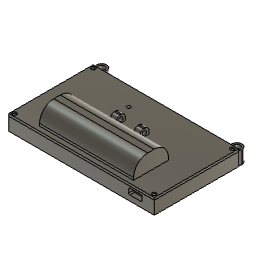
OS_EINK_CAD (Autodesk Fusion 360 design; units mm, degrees)
Autodesk Fusion 360 part; units mm, degrees
sketch "Sketch1" plane through (0, 0, 0) normal (0, 0, 1) x (1, 0, 0)
  line L0 (0, 0) -> (114, 0)
  line L1 (0, 0) -> (0, 63)
  line L2 (0, 63) -> (114, 63)
  line L3 (114, 0) -> (114, 63)
  dimension "d1" = 114
  dimension "d2" = 63
  constraint coincident L0.start L1.start
  constraint horizontal L0
  constraint perpendicular L0 L1
  constraint perpendicular L1 L2
  constraint coincident L2 L3.end
  constraint perpendicular L2 L3
  measures "d1" distance of L0.start L0.end
  measures "d2" distance of L0.start L1.end
extrude "Extrude1" add sketch "Sketch1" along normal blind 4 makes body 1
sketch "Sketch2" plane through (0, 0, 4) normal (0, 0, 1) x (-1, 0, 0)
  line L0 (0, 0) -> (-114, 0)
  line L1 (-114, 0) -> (-114, -63)
  line L2 (-114, -63) -> (0, -63)
  line L3 (0, -63) -> (0, 0)
  line L4 (-20, -3) -> (-20, -25.0318)
  line L5 (-20, -25.0318) -> (-85, -25.0318)
  line L6 (-20, -25.0318) -> (-93.9139, -25.0318)
  line L7 (-93.9139, -25.0318) -> (-93.9139, -1.7356)
  line L8 (-93.9139, -1.7356) -> (-20, -1.7356)
  line L9 (-20, -1.7356) -> (-20, -25.0318)
  constraint perpendicular L4 L5
  constraint horizontal L6
  constraint vertical L7
  constraint horizontal L8
  constraint vertical L9
extrude "Extrude2" add sketch "Sketch2" along normal blind 17 separate body contours L4 L5 L6 L7 L8 L9 makes body 2
sketch "Sketch3" plane through (0, 0, 4) normal (0, 0, 1) x (-1, 0, 0)
  line L0 (0, 0) -> (-114, 0)
  line L1 (-114, 0) -> (-114, -63)
  line L2 (-114, -63) -> (0, -63)
  line L3 (0, -63) -> (0, 0)
  line L4 (-108, -53.9996) -> (-108, -32)
  line L5 (-108, -32) -> (-14.4334, -32)
  line L6 (-14.4334, -32) -> (-14.4334, -63)
  line L7 (-14.4334, -63) -> (-108, -63)
  line L8 (-108, -63) -> (-108, -32)
  constraint horizontal L5
  constraint vertical L6
  constraint horizontal L7
  constraint vertical L8
  constraint coincident L2 L6.end
extrude "Extrude1'" add sketch "Sketch3" along normal blind 8.4 separate body contours L2 L4 L5 L6 L7 L8 makes body 3 in component "Case"
copy_body "CutPasteBodies1" bodies 3 removing the originals makes body 4
sketch "Sketch4" plane through (0, 0, 4) normal (0, 0, 1) x (-1, 0, 0)
  line L0 (0, 0) -> (-114, 0)
  line L1 (-114, 0) -> (-114, -63)
  line L2 (-114, -63) -> (0, -63)
  line L3 (0, -63) -> (0, 0)
  line L4 (-109.5, 0) -> (-109.5, -7.5)
  line L5 (-109.5, -7.5) -> (-100.2, -7.5)
  line L6 (-100.2, -7.5) -> (-100.2, 0)
  line L7 (-100.2, 0) -> (-109.5, 0)
  dimension "d19" = 7.5
  dimension "d20" = 9.3
  constraint coincident L0 L4.start
  constraint perpendicular L4 L5
  constraint coincident L0 L6.end
  constraint perpendicular L0 L6
  measures "d19" distance of L4.start L4.end
  measures "d20" distance of L4.end L5.end
extrude "Extrude3" add sketch "Sketch4" along normal blind 7.4 separate body contours L0 L4 L5 L6 L7 makes body 5
sketch "Sketch5" plane through (0, 0, 0) normal (0, 0, -1) x (1, 0, 0)
  line L0 (114, 0) -> (0, 0)
  line L1 (0, 0) -> (0, -63)
  line L2 (0, -63) -> (114, -63)
  line L3 (114, -63) -> (114, 0)
  line L4 (2.053, -1.9988) -> (111.9324, -1.9988)
  line L5 (111.9324, -1.9988) -> (111.9324, -60.7463)
  line L6 (111.9324, -60.7463) -> (2.053, -60.7463)
  line L7 (2.053, -60.7463) -> (2.053, -1.9988)
  line L8 (-3.2421, 3.0422) -> (117.6071, 3.0422)
  line L9 (117.6071, 3.0422) -> (117.6071, -66.157)
  line L10 (117.6071, -66.157) -> (-3.2421, -66.157)
  line L11 (-3.2421, -66.157) -> (-3.2421, 3.0422)
  constraint horizontal L4
  constraint vertical L5
  constraint horizontal L6
  constraint vertical L7
  constraint horizontal L8
  constraint vertical L9
  constraint horizontal L10
  constraint vertical L11
extrude "Extrude4" add sketch "Sketch5" along normal blind 2 separate body contours L0 L1 L2 L3 | L8 L9 L10 L11 makes body 6
copy_body "CutPasteBodies1'" bodies 6 removing the originals makes body 7 in component "Case"
sketch "Sketch6" plane through (0, 0, 0) normal (0, 0, 1) x (-1, 0, 0)
  line L0 (-2.053, -60.7463) -> (-111.9324, -60.7463)
  line L1 (-111.9324, -60.7463) -> (-111.9324, -1.9988)
  line L2 (-111.9324, -1.9988) -> (-2.053, -1.9988)
  line L3 (-2.053, -1.9988) -> (-2.053, -60.7463)
  line L4 (-117.6071, -66.157) -> (3.2421, -66.157)
  line L5 (3.2421, -66.157) -> (3.2421, 3.0422)
  line L6 (3.2421, 3.0422) -> (-117.6071, 3.0422)
  line L7 (-117.6071, 3.0422) -> (-117.6071, -66.157)
  line L8 (0.1598, -63.129) -> (-114.0751, -63.129)
  line L9 (-114.0751, -63.129) -> (-114.0751, 0.0707)
  line L10 (-114.0751, 0.0707) -> (0.1598, 0.0707)
  line L11 (0.1598, 0.0707) -> (0.1598, -63.129)
  line L12 (3.2421, -66.157) -> (-117.6071, -66.157)
  line L13 (-117.6071, -66.157) -> (-117.6071, 3.0422)
  line L14 (-117.6071, 3.0422) -> (3.2421, 3.0422)
  line L15 (3.2421, 3.0422) -> (3.2421, -66.157)
  constraint horizontal L8
  constraint vertical L9
  constraint horizontal L10
  constraint vertical L11
  constraint horizontal L12
  constraint vertical L13
  constraint horizontal L14
  constraint vertical L15
  constraint coincident L6.end L7.start
  constraint coincident L4.end L5.start
extrude "Extrude2'" add sketch "Sketch6" along normal blind 9 contours L4 L5 L6 L7 L12 L13 L14 L15 bodies 7 in component "Case"
sketch "Sketch7" plane through (0, 0, 9) normal (0, 0, 1) x (-1, 0, 0)
  line L0 (-114.0751, 0.0707) -> (0.1598, 0.0707)
  line L1 (0.1598, 0.0707) -> (0.1598, -63.129)
  line L2 (0.1598, -63.129) -> (-114.0751, -63.129)
  line L3 (-114.0751, -63.129) -> (-114.0751, 0.0707)
  line L4 (3.2421, 3.0422) -> (-117.6071, 3.0422)
  line L5 (-117.6071, 3.0422) -> (-117.6071, -66.157)
  line L6 (-117.6071, -66.157) -> (3.2421, -66.157)
  line L7 (3.2421, -66.157) -> (3.2421, 3.0422)
  line L8 (0.1598, -9.803) -> (1.5167, -9.803)
  line L9 (1.5167, -9.803) -> (1.5167, -57.1457)
  line L10 (1.5167, -57.1457) -> (0.1598, -57.1457)
  line L11 (0.1598, -57.1457) -> (0.1598, -9.803)
  constraint horizontal L8
  constraint vertical L9
  constraint horizontal L10
  constraint vertical L11
  constraint coincident L1 L8.start
extrude "Extrude3'" cut sketch "Sketch7" against normal blind 9 contours L1 L8 L9 L10 L11 bodies 7 in component "Case"
sketch "Sketch8" plane through (0, -3.0422, 0) normal (0, -1, 0) x (1, 0, 0)
  line L0 (-3.2421, 9) -> (-3.2421, -2)
  line L1 (-3.2421, -2) -> (117.6071, -2)
  line L2 (117.6071, -2) -> (117.6071, 9)
  line L3 (117.6071, 9) -> (-3.2421, 9)
  line L4 (96.9453, 7.5501) -> (108.2199, 7.5501)
  line L5 (108.2199, 7.5501) -> (108.2199, 2.4633)
  line L6 (108.2199, 2.4633) -> (96.9453, 2.4633)
  line L7 (96.9453, 2.4633) -> (96.9453, 7.5501)
  constraint horizontal L4
  constraint vertical L5
  constraint horizontal L6
  constraint vertical L7
extrude "Extrude4'" cut sketch "Sketch8" against normal blind 3 contours L4 L5 L6 L7 bodies 7 in component "Case"
extrude "Extrude5" cut 1 faces at (45.6223, 49.6665, 12.4) along direction (0, 0, -1) blind 4 on bodies 4 bodies 4
extrude "Extrude6" cut 1 faces at (106.4, 2.5, 11.4) along direction (0, 0, -1) blind 4 on bodies 5 bodies 5
sketch "Sketch9" plane through (0, 0, 9) normal (0, 0, 1) x (-1, 0, 0)
  line L0 (1.5167, -57.1457) -> (0.1598, -57.1457)
  line L1 (0.1598, -57.1457) -> (0.1598, -63.129)
  line L2 (0.1598, -63.129) -> (-114.0751, -63.129)
  line L3 (-114.0751, -63.129) -> (-114.0751, 0.0707)
  line L4 (-114.0751, 0.0707) -> (0.1598, 0.0707)
  line L5 (0.1598, 0.0707) -> (0.1598, -9.803)
  line L6 (0.1598, -9.803) -> (1.5167, -9.803)
  line L7 (1.5167, -9.803) -> (1.5167, -57.1457)
  line L8 (3.2421, 3.0422) -> (-117.6071, 3.0422)
  line L9 (-117.6071, 3.0422) -> (-117.6071, -66.157)
  line L10 (-117.6071, -66.157) -> (3.2421, -66.157)
  line L11 (3.2421, -66.157) -> (3.2421, 3.0422)
  circle A0 through (2.8751, 1.1502, 3) (0.6251, 2.4493, 3) (0.6251, -0.1488, 3)
  circle A1 through (-114.6218, 1.1732, 3) (-116.1218, 2.0393, 3) (-116.1218, 0.3072, 3)
  circle A2 through (-114.773, -64.2526, 3) (-116.273, -63.3865, 3) (-116.273, -65.1186, 3)
  circle A3 through (2.385, -64.4488, 3) (0.885, -63.5828, 3) (0.885, -65.3148, 3)
  point P0 (1.3751, 1.1502)
  dimension "d40" = 3
  dimension "d41" = 2
  dimension "d42" = 2
  dimension "d43" = 2
sketch "Sketch10" plane through (0, 0, 9) normal (0, 0, 1) x (-1, 0, 0)
sketch "Sketch11" plane through (0, 0, 9) normal (0, 0, 1) x (-1, 0, 0)
  line L0 (3.2373, 3.0256) -> (-117.6011, 3.0256)
  line L1 (-117.6011, 3.0256) -> (-117.6011, -66.1556)
  line L2 (-117.6011, -66.1556) -> (3.2373, -66.1556)
  line L3 (3.2373, -66.1556) -> (3.2373, 3.0256)
  constraint horizontal L0
  constraint vertical L1
  constraint horizontal L2
  constraint vertical L3
extrude "Extrude7" add sketch "Sketch11" along normal blind 3 separate body makes body 8
copy_body "CutPasteBodies2" bodies 8 removing the originals makes body 9 in component "Case"
sketch "Sketch12" plane through (0, 0, 12) normal (0, 0, 1) x (-1, 0, 0)
  line L0 (3.2373, -66.1556) -> (3.2373, 3.0256)
  line L1 (3.2373, 3.0256) -> (-117.6011, 3.0256)
  line L2 (-117.6011, 3.0256) -> (-117.6011, -66.1556)
  line L3 (-117.6011, -66.1556) -> (3.2373, -66.1556)
  line L4 (-17.965, -29.1961) -> (-97.3004, -29.1961)
  line L5 (-97.3004, -29.1961) -> (-97.3004, 0.2524)
  line L6 (-97.3004, 0.2524) -> (-17.965, 0.2524)
  line L7 (-17.965, 0.2524) -> (-17.965, -29.1961)
  constraint horizontal L4
  constraint vertical L5
  constraint horizontal L6
  constraint vertical L7
extrude "Extrude5'" add sketch "Sketch12" along normal blind 14 separate body contours L4 L5 L6 L7 makes body 10 in component "Case"
sketch "Sketch13" plane through (0, 0, 12) normal (0, 0, 1) x (1, 0, 0)
sketch "Sketch14" plane through (0, 63.129, 0) normal (0, -1, 0) x (1, 0, 0)
  line L0 (-0.1598, 0) -> (114.0751, 0)
  line L1 (114.0751, 0) -> (114.0751, 9)
  line L2 (114.0751, 9) -> (-0.1598, 9)
  line L3 (-0.1598, 9) -> (-0.1598, 0)
sketch "Sketch15" plane through (0, 66.157, 0) normal (0, 1, 0) x (-1, 0, 0)
  line L0 (-117.6071, 9) -> (-117.6071, -2)
  line L1 (-117.6071, -2) -> (3.2421, -2)
  line L2 (3.2421, -2) -> (3.2421, 9)
  line L3 (3.2421, 9) -> (-117.6071, 9)
sketch "Sketch16" plane through (0, 66.157, 0) normal (0, 1, 0) x (-1, 0, 0)
  line L0 (-94.6954, 3.5982) -> (-47.0974, 3.5982)
  line L1 (-47.0974, 3.5982) -> (-47.0974, 0.7193)
  line L2 (-47.0974, 0.7193) -> (-94.6954, 0.7193)
  line L3 (-94.6954, 0.7193) -> (-94.6954, 3.5982)
  constraint horizontal L0
  constraint vertical L1
  constraint horizontal L2
  constraint vertical L3
sketch "Sketch18" plane through (0, 0, 9) normal (0, 0, 1) x (-1, 0, 0)
  line L0 (1.5167, -57.1457) -> (0.1598, -57.1457)
  line L1 (0.1598, -57.1457) -> (0.1598, -63.129)
  line L2 (0.1598, -63.129) -> (-114.0751, -63.129)
  line L3 (-114.0751, -63.129) -> (-114.0751, 0.0707)
  line L4 (-114.0751, 0.0707) -> (0.1598, 0.0707)
  line L5 (0.1598, 0.0707) -> (0.1598, -9.803)
  line L6 (0.1598, -9.803) -> (1.5167, -9.803)
  line L7 (1.5167, -9.803) -> (1.5167, -57.1457)
  line L8 (3.2421, 3.0422) -> (-117.6071, 3.0422)
  line L9 (-117.6071, 3.0422) -> (-117.6071, -66.157)
  line L10 (-117.6071, -66.157) -> (3.2421, -66.157)
  line L11 (3.2421, -66.157) -> (3.2421, 3.0422)
  line L12 (-96.1619, -63.129) -> (-45.1217, -63.129)
  line L13 (-45.1217, -63.129) -> (-45.1217, -64.3836)
  line L14 (-45.1217, -64.3836) -> (-96.1619, -64.3836)
  line L15 (-96.1619, -64.3836) -> (-96.1619, -63.129)
  constraint horizontal L12
  constraint vertical L13
  constraint horizontal L14
  constraint vertical L15
  constraint coincident L2 L12.start
extrude "Extrude10" cut sketch "Sketch18" against normal blind 9 contours L2 L12 L13 L14 L15 bodies 7 in component "Case"
extrude "Extrude11" cut 1 faces at (77.3217, 20.0348, 9) along direction (0, 0, 1) blind 1 on bodies 9 bodies 9 10 in component "Case"
move_body "Move1" bodies 10 9 to x (1, 0, 0) y (0, 1, 0) z (0, 0, 1) at (0, 0, -1) in component "Case"
fillet "Fillet3" radius 12 1 edges at (57.6327, -0.2524, 25) on bodies 10 in component "Case"
fillet "Fillet4" radius 12 1 edges at (57.6327, 29.1961, 25) on bodies 10 in component "Case"
shell "Shell2" thickness 1 removed faces 1 at (44.4101, 19.3799, 11) on bodies 10 in component "Case"
sketch "Sketch19" plane through (0, 0, 11) normal (0, 0, -1) x (1, 0, 0)
  line L0 (18.965, -28.1961) -> (18.965, -0.7476)
  line L1 (18.965, -0.7476) -> (96.3004, -0.7476)
  line L2 (96.3004, -0.7476) -> (96.3004, -28.1961)
  line L3 (96.3004, -28.1961) -> (18.965, -28.1961)
  line L4 (97.3004, 0.2524) -> (17.965, 0.2524)
  line L5 (17.965, 0.2524) -> (17.965, -29.1961)
  line L6 (17.965, -29.1961) -> (97.3004, -29.1961)
  line L7 (97.3004, -29.1961) -> (97.3004, 0.2524)
  line L8 (18.965, -28.1961) -> (96.3004, -28.1961)
  line L9 (96.3004, -28.1961) -> (96.3004, -0.7476)
  line L10 (96.3004, -0.7476) -> (18.965, -0.7476)
  line L11 (18.965, -0.7476) -> (18.965, -28.1961)
  constraint horizontal L8
  constraint vertical L9
  constraint horizontal L10
  constraint vertical L11
  constraint coincident L1.end L2.start
  constraint coincident L0.start L3.end
extrude "Extrude12" cut sketch "Sketch19" along normal blind 44 contours L0 L1 L2 L3 L8 L9 L10 L11 bodies 9 in component "Case"
extrude "Extrude13" add 1 faces at (44.7434, 28.8628, 11) along direction (0, 0, -1) blind 0.1 on bodies 10 bodies 10 9 in component "Case"
extrude "Extrude14" add 1 faces at (117.6071, 43.0906, 5.3333) along direction (1, 0, 0) blind 1 on bodies 7 bodies 7 in component "Case"
extrude "Extrude15" add sketch "Sketch15" along normal blind 1 bodies 7 in component "Case"
extrude "Extrude16" add 1 faces at (117.9404, 66.157, 5.3333) along direction (0, 1, 0) blind 1 on bodies 7 bodies 7 in component "Case"
extrude "Extrude17" add 1 faces at (30.1537, -3.0422, 3.1544) along direction (0, -1, 0) blind 1 on bodies 7 bodies 7 in component "Case"
extrude "Extrude19" add 1 faces at (-3.2421, 19.6909, 5.3333) along direction (-1, 0, 0) blind 1 on bodies 7 bodies 7 in component "Case"
extrude "Extrude20" add 1 faces at (77.3217, 66.1556, 9.6667) along direction (0, 1, 0) blind 1 on bodies 10 bodies 10 in component "Case"
extrude "Extrude21" add 1 faces at (-3.2373, 43.7618, 10.3333) along direction (-1, 0, 0) blind 1 on bodies 10 bodies 10 in component "Case"
extrude "Extrude22" add 1 faces at (36.3755, -3.0256, 10.3333) along direction (0, -1, 0) blind 1 on bodies 10 bodies 10 in component "Case"
extrude "Extrude23" add 1 faces at (117.6011, 19.7014, 10.3333) along direction (1, 0, 0) blind 1 on bodies 10 bodies 10 in component "Case"
hole "Hole2" at (41.6318, 51.3598, 11) direction (0, 0, -1) diameter 3 depth 5 tip angle 180 bodies 10 in component "Case"
sketch "Sketch20" plane through (0, 0, 11) normal (0, 0, 1) x (-1, 0, 0)
  circle A0 centre (-41.6318, -51.3598) radius 1.5
  line L0 (-118.6011, -67.1556) -> (4.2373, -67.1556)
  line L1 (4.2373, -67.1556) -> (4.2373, 4.0256)
  line L2 (4.2373, 4.0256) -> (-118.6011, 4.0256)
  line L3 (-118.6011, 4.0256) -> (-118.6011, -67.1556)
  line L4 (-17.965, 0.2524) -> (-17.965, -29.1961)
  line L5 (-17.965, -29.1961) -> (-97.3004, -29.1961)
  line L6 (-97.3004, -29.1961) -> (-97.3004, 0.2524)
  line L7 (-97.3004, 0.2524) -> (-17.965, 0.2524)
  circle A1 centre (1.7264, 1.6861) radius 1.5
  circle A2 centre (1.6398, -64.7578) radius 1.5
  circle A3 centre (-115.8829, 1.4876) radius 1.5
  circle A4 centre (-115.9786, -64.5367) radius 1.5
  dimension "d107" = 3
  dimension "d108" = 3
  dimension "d109" = 3
  dimension "d110" = 3
  measures "d107" diameter of A1
  measures "d108" diameter of A2
  measures "d109" diameter of A3
  measures "d110" diameter of A4
hole "Hole4" at (-1.7264, -1.6861, 11) at (-1.6398, 64.7578, 11) at (115.9786, 64.5367, 11) at (115.8829, -1.4876, 11) direction (0, 0, -1) diameter 2.4 depth 6 tip angle 180 countersink diameter 3.5 countersink angle 90 bodies 7 10 in component "Case"
fillet "Fillet5" radius 1 1 edges at (108.2199, -2.0565, 2.4633) on bodies 7 in component "Case"
fillet "Fillet6" radius 1 1 edges at (96.9453, -2.0565, 2.4633) on bodies 7 in component "Case"
fillet "Fillet7" radius 1 1 edges at (96.9453, -2.0565, 7.5501) on bodies 7 in component "Case"
fillet "Fillet8" radius 1 1 edges at (108.2199, -2.0565, 7.5501) on bodies 7 in component "Case"
sketch "Sketch21" plane through (0, -0.0707, 0) normal (0, 1, 0) x (-1, 0, 0)
  line L0 (-108.2199, 3.4633) -> (-108.2199, 6.5501)
  arc A0 (-107.2199, 7.5501) -> (-108.2199, 6.5501) centre (-107.2199, 6.5501) ccw
  line L1 (-107.2199, 7.5501) -> (-97.9453, 7.5501)
  arc A1 (-96.9453, 6.5501) -> (-97.9453, 7.5501) centre (-97.9453, 6.5501) ccw
  line L2 (-96.9453, 6.5501) -> (-96.9453, 3.4633)
  arc A2 (-97.9453, 2.4633) -> (-96.9453, 3.4633) centre (-97.9453, 3.4633) ccw
  line L3 (-97.9453, 2.4633) -> (-107.2199, 2.4633)
  arc A3 (-108.2199, 3.4633) -> (-107.2199, 2.4633) centre (-107.2199, 3.4633) ccw
  line L4 (-114.0751, 0) -> (0.1598, 0)
  line L5 (0.1598, 0) -> (0.1598, 9)
  line L6 (0.1598, 9) -> (-114.0751, 9)
  line L7 (-114.0751, 9) -> (-114.0751, 0)
extrude "Extrude24" add 1 faces at (2.053, 41.1638, -0.6667) along direction (1, 0, 0) blind 6 on bodies 7 bodies 7 in component "Case"
extrude "Extrude25" add 1 faces at (8.053, 41.1638, -0.6667) along direction (1, 0, 0) blind 2.5 on bodies 7 bodies 7 in component "Case"
extrude "Extrude26" add 1 faces at (44.3461, 1.9988, -1.3333) along direction (0, 1, 0) blind 1.5 on bodies 7 bodies 7 in component "Case"
extrude "Extrude27" add 1 faces at (78.1393, 60.7463, -1.3333) along direction (0, -1, 0) blind 1.5 on bodies 7 bodies 7 in component "Case"
extrude "Extrude28" add 1 faces at (111.9324, 22.0813, -0.6667) along direction (-1, 0, 0) blind 1.5 on bodies 7 bodies 7 in component "Case"
sketch "Sketch24" plane through (0, 67.157, 0) normal (0, 1, 0) x (-1, 0, 0)
  line L0 (4.2421, 9) -> (-118.6071, 9)
  line L1 (-118.6071, 9) -> (-118.6071, -2)
  line L2 (-118.6071, -2) -> (4.2421, -2)
  line L3 (4.2421, -2) -> (4.2421, 9)
  line L4 (4.2421, -2) -> (-10.4083, -2)
  line L5 (-10.4083, -2) -> (-10.4083, 0.5)
  line L6 (-10.4083, 0.5) -> (4.2421, 0.5)
  line L7 (4.2421, 0.5) -> (4.2421, -2)
  line L8 (-118.6071, -2) -> (-110.8528, -2)
  line L9 (-110.8528, -2) -> (-110.8528, 0.5)
  line L10 (-110.8528, 0.5) -> (-118.6071, 0.5)
  line L11 (-118.6071, 0.5) -> (-118.6071, -2)
  dimension "d138" = 2.5
  dimension "d139" = 2.5
  constraint horizontal L4
  constraint vertical L5
  constraint horizontal L6
  constraint vertical L7
  constraint coincident L2.end L3.start
  constraint horizontal L8
  constraint vertical L9
  constraint horizontal L10
  constraint vertical L11
  constraint coincident L1.end L2.start
  measures "d138" distance of L2.end L6.end
  measures "d139" distance of L1.end L10.end
extrude "Extrude31" add sketch "Sketch24" along normal blind 10 contours L2 L3 L4 L5 L6 L7 | L1 L2 L8 L9 L10 L11 bodies 7 in component "Case"
sketch "Sketch25" plane through (0, 0, -2) normal (0, 0, -1) x (1, 0, 0)
  line L0 (110.4324, -59.2463) -> (10.553, -59.2463)
  line L1 (10.553, -59.2463) -> (10.553, -3.4988)
  line L2 (10.553, -3.4988) -> (110.4324, -3.4988)
  line L3 (110.4324, -3.4988) -> (110.4324, -59.2463)
  line L4 (118.6071, -77.157) -> (118.6071, 4.0422)
  line L5 (118.6071, 4.0422) -> (-4.2421, 4.0422)
  line L6 (-4.2421, 4.0422) -> (-4.2421, -77.157)
  line L7 (-4.2421, -77.157) -> (10.4083, -77.157)
  line L8 (10.4083, -77.157) -> (10.4083, -67.157)
  line L9 (10.4083, -67.157) -> (110.8528, -67.157)
  line L10 (110.8528, -67.157) -> (110.8528, -77.157)
  line L11 (110.8528, -77.157) -> (118.6071, -77.157)
  circle A0 centre (-0.0244, -70.1431) radius 4.2172
  line L12 (10.4083, -67.157) -> (-4.2421, -67.157)
  line L13 (-4.2421, -67.157) -> (-4.2421, -65.1413)
  line L14 (-4.2421, -65.1413) -> (10.4083, -65.1413)
  line L15 (10.4083, -65.1413) -> (10.4083, -67.157)
  line L16 (10.4083, -67.157) -> (3.0831, -77.157)
  line L17 (3.0831, -77.157) -> (-4.2421, -67.157)
  line L18 (3.1249, -74.3509) -> (8.3946, -67.157)
  line L19 (3.1249, -74.3509) -> (-2.1448, -67.157)
  circle A1 centre (-0.0244, -70.1431) radius 1.7097
  line L20 (3.0831, -72.974) -> (7.3442, -67.157)
  line L21 (3.0831, -72.974) -> (-1.2088, -67.115)
  line L22 (3.0831, -72.1297) -> (6.7257, -67.157)
  line L23 (3.0831, -72.1297) -> (-0.5595, -67.157)
  line L24 (-4.0558, -67.157) -> (-4.0558, -70.1199)
  line L25 (-4.0558, -70.1199) -> (-4.2421, -70.1199)
  constraint horizontal L12
  constraint vertical L13
  constraint horizontal L14
  constraint vertical L15
  constraint coincident L6 L13.end
  constraint coincident L8.end L9.start
  constraint midpoint L7 L16.end
  constraint coincident L12 L18.end
  constraint parallel L16 L18
  constraint coincident L12 L19.end
  constraint parallel L17 L19
  constraint coincident L12 L20.end
  constraint parallel L18 L20
  constraint parallel L19 L21
  constraint coincident L12 L22.end
  constraint parallel L20 L22
  constraint coincident L12 L23.end
  constraint parallel L21 L23
  constraint coincident L12 L24.start
  constraint perpendicular L12 L24
  constraint coincident L6 L25.end
  constraint perpendicular L6 L25
sketch "Sketch26" plane through (0, 0, -2) normal (0, 0, -1) x (1, 0, 0)
  line L0 (110.4324, -59.2463) -> (10.553, -59.2463)
  line L1 (10.553, -59.2463) -> (10.553, -3.4988)
  line L2 (10.553, -3.4988) -> (110.4324, -3.4988)
  line L3 (110.4324, -3.4988) -> (110.4324, -59.2463)
  line L4 (118.6071, -77.157) -> (118.6071, 4.0422)
  line L5 (118.6071, 4.0422) -> (-4.2421, 4.0422)
  line L6 (-4.2421, 4.0422) -> (-4.2421, -77.157)
  line L7 (-4.2421, -77.157) -> (10.4083, -77.157)
  line L8 (10.4083, -77.157) -> (10.4083, -67.157)
  line L9 (10.4083, -67.157) -> (110.8528, -67.157)
  line L10 (110.8528, -67.157) -> (110.8528, -77.157)
  line L11 (110.8528, -77.157) -> (118.6071, -77.157)
  circle A0 centre (113.5421, -71.1591) radius 2.9925
  circle A1 centre (113.5421, -71.1591) radius 5.0661
  line L12 (10.4083, -67.157) -> (106.5, -67.157)
  line L13 (109.6276, -67.157) -> (118.6071, -67.157)
  constraint concentric A0 A1
  constraint coincident L8.end L9.start
  constraint perpendicular L6 L12
  constraint coincident L9 L13.start
  constraint coincident L4 L13.end
  constraint perpendicular L4 L13
sketch "Sketch28" plane through (0, 0, -2) normal (0, 0, -1) x (1, 0, 0)
sketch "Sketch27" plane through (0, 0, -2) normal (0, 0, -1) x (1, 0, 0)
extrude "Extrude35" add 1 faces at (113.4376, 70.4903, 0.5) along direction (0, 0, 1) blind 1 on bodies 7 bodies 7 in component "Case"
extrude "Extrude36" cut sketch "Sketch25" against normal blind 4.5 contours A0 L12 L16 L17 L18 L19 | L7 L8 L16 | A0 L12 L18 L19 L20 | L6 L7 A0 L17 | A0 L12 L20 L22 | A0 L12 L22 | L17 A1 | L17 L19 A1 | L19 A1 L21 | A1 L21 L23 | A1 L23 bodies 7 in component "Case"
sketch "Sketch29" plane through (0, 0, -2) normal (0, 0, -1) x (1, 0, 0)
  circle A0 centre (114.3946, -70.0022) radius 1.7117
  circle A1 centre (114.3946, -70.0022) radius 4.214
  line L0 (110.85, -67.15) -> (118.6746, -67.15)
  line L1 (118.5961, -77.1217) -> (110.85, -77.1217)
  line L2 (110.85, -77.1217) -> (110.85, -67.15)
  line L3 (110.85, -67.15) -> (118.5961, -67.15)
  line L4 (118.5961, -67.15) -> (118.5961, -77.1217)
  line L5 (119.1605, -77.7264) -> (110.5352, -77.7264)
  line L6 (110.5352, -77.7264) -> (110.5352, -67.15)
  line L7 (110.5352, -67.15) -> (119.1605, -67.15)
  line L8 (119.1605, -67.15) -> (119.1605, -77.7264)
  line L9 (110.919, -72.385) -> (110.919, -67.6194)
  constraint concentric A0 A1
  constraint horizontal L0
  constraint horizontal L1
  constraint vertical L2
  constraint horizontal L3
  constraint vertical L4
  constraint horizontal L5
  constraint vertical L6
  constraint horizontal L7
  constraint vertical L8
  constraint coincident A1 L9.start
  constraint coincident A1 L9.end
  constraint perpendicular L0 L9
extrude "Extrude41" add sketch "Sketch29" against normal blind 3.5 contours A1 L2 L9 | A1 L2 L6 | A1 L6 bodies 7 in component "Case"
extrude "Extrude40" cut sketch "Sketch29" against normal blind 6 contours A0 | A1 L0 L1 L2 L4 L5 L6 L7 L8 | A1 L0 L3 L4 L7 | A1 L1 L2 L4 | A1 L0 L2 L3 L7 bodies 7 in component "Case"
extrude "Extrude42" add 1 faces at (110.85, 67.1546, 0) along direction (1, 0, 0) blind 0.45 on bodies 7 bodies 7 in component "Case"
extrude "Extrude44" add 1 faces at (118.239, 67.1546, 4) along direction (0, 0, -1) blind 6 on bodies 7 bodies 7 in component "Case"
extrude "Extrude45" cut sketch "Sketch25" against normal blind 6 contours L6 A0 L17 L24 | L12 L17 L24 | A0 L12 L17 L24 | A0 L17 L24 bodies 7 in component "Case"
extrude "Extrude46" add 1 faces at (-0.067, 67.584, 0.5) along direction (0, 0, 1) blind 9 on bodies 7 bodies 7 in component "Case"
extrude "Extrude47" add 1 faces at (114.3519, 67.5364, 1.5) along direction (0, 0, 1) blind 7.5 on bodies 7 bodies 7 in component "Case"
sketch "Sketch31" plane through (0, 0, -2) normal (0, 0, -1) x (1, 0, 0)
  arc A0 (-3.0023, -67.157) -> (2.9535, -67.157) centre (-0.0244, -70.1431) ccw
  line L0 (2.9535, -67.157) -> (111.2862, -67.157)
  arc A1 (111.2862, -67.157) -> (118.6071, -70.1137) centre (114.3946, -70.0022) ccw
  line L1 (118.6071, -70.1137) -> (118.6071, -69.8908)
  arc A2 (118.6071, -69.8908) -> (117.503, -67.157) centre (114.3946, -70.0022) ccw
  line L2 (117.503, -67.157) -> (118.6071, -67.157)
  line L3 (118.6071, -67.157) -> (118.6071, 4.0422)
  line L4 (118.6071, 4.0422) -> (-4.2421, 4.0422)
  line L5 (-4.2421, 4.0422) -> (-4.2421, -67.157)
  line L6 (-4.2421, -67.157) -> (-3.0023, -67.157)
  circle A3 centre (-0.0244, -70.1431) radius 1.7097
  line L7 (110.4324, -59.2463) -> (10.553, -59.2463)
  line L8 (10.553, -59.2463) -> (10.553, -3.4988)
  line L9 (10.553, -3.4988) -> (110.4324, -3.4988)
  line L10 (110.4324, -3.4988) -> (110.4324, -59.2463)
  circle A4 centre (114.3946, -70.0022) radius 1.7117
  circle A5 centre (-0.0244, -70.1431) radius 2.6211
  circle A6 centre (114.3946, -70.0022) radius 2.621
  dimension "d176" = 5.242
  constraint concentric A0 A5
  constraint concentric A1 A6
  measures "d176" diameter of A6
extrude "Extrude48" cut sketch "Sketch31" against normal blind 11 contours A5 | A6 bodies 7 in component "Case"
extrude "Extrude49" cut 1 faces at (-2.0043, 68.9508, 9) along direction (0, 0, 1) blind 3 on bodies 7 bodies 7 in component "Case"
sketch "Sketch32" plane through (0, 0, 9) normal (0, 0, 1) x (-1, 0, 0)
  line L0 (0, 0) -> (-15, 0)
  line L1 (-15, 0) -> (-15, -1)
  line L2 (-15, -1) -> (0, -1)
  line L3 (0, -1) -> (0, 0)
  constraint horizontal L0
  constraint vertical L1
  constraint horizontal L2
  constraint vertical L3
  constraint coincident L0.start L3.end
extrude "Extrude50" add sketch "Sketch32" along normal blind -9 and the other way blind -1 bodies 7 in component "Case"
extrude "Extrude51" cut 1 faces at (10, 0.3333, 10) along direction (0, 0, -1) blind 9 on bodies 7 bodies 7 in component "Case"
sketch "Sketch33" plane through (0, 0, 9) normal (0, 0, 1) x (-1, 0, 0)
  line L0 (-10.5, -1) -> (0, -1)
  line L1 (0, -1) -> (0, 0)
  line L2 (0, 0) -> (-10.5, 0)
  line L3 (-10.5, 0) -> (-10.5, -1)
  constraint horizontal L0
  constraint vertical L1
  constraint horizontal L2
  constraint vertical L3
  constraint coincident L1.end L2.start
extrude "Extrude52" cut sketch "Sketch33" against normal blind 9 bodies 7 in component "Case"
extrude "Extrude53" cut 1 faces at (13.5, 1, 0.6667) along direction (0, -1, 0) blind 0.5 on bodies 7 bodies 7 in component "Case"
extrude "Extrude54" add 1 faces at (13.5, 0.1667, 1) along direction (0, 0, 1) blind 1 on bodies 7 bodies 7 in component "Case"
sketch "Sketch34" plane through (0, 0, 11) normal (0, 0, 1) x (-1, 0, 0)
  circle A0 centre (-115.9786, -64.5367) radius 1.75
  circle A1 centre (1.7264, 1.6861) radius 1.75
  circle A2 centre (1.6398, -64.7578) radius 1.75
  circle A3 centre (-115.8829, 1.4876) radius 1.75
  circle A4 centre (-41.6318, -51.3598) radius 1.5
  line L0 (-118.6011, -67.1556) -> (4.2373, -67.1556)
  line L1 (4.2373, -67.1556) -> (4.2373, 4.0256)
  line L2 (4.2373, 4.0256) -> (-118.6011, 4.0256)
  line L3 (-118.6011, 4.0256) -> (-118.6011, -67.1556)
  line L4 (-17.965, 0.2524) -> (-17.965, -29.1961)
  line L5 (-17.965, -29.1961) -> (-97.3004, -29.1961)
  line L6 (-97.3004, -29.1961) -> (-97.3004, 0.2524)
  line L7 (-97.3004, 0.2524) -> (-17.965, 0.2524)
  line L8 (-55, -40) -> (-60.2654, -40)
  line L9 (-60.2654, -40) -> (-60.2654, -32.5385)
  line L10 (-60.2654, -32.5385) -> (-55, -32.5385)
  line L11 (-55, -32.5385) -> (-55, -40)
  line L12 (-55, -40) -> (-60.2654, -32.5385) construction
  line L13 (-60.2654, -40) -> (-55, -32.5385) construction
  point P0 (-57.6327, -36.2693)
  constraint horizontal L8
  constraint perpendicular L8 L9
  constraint parallel L8 L10
  constraint parallel L9 L11
  constraint coincident L12 P0
  constraint coincident L13 P0
sketch "Sketch35" plane through (0, 0, 11) normal (0, 0, 1) x (-1, 0, 0)
  circle A0 centre (-115.9786, -64.5367) radius 1.75
  circle A1 centre (1.7264, 1.6861) radius 1.75
  circle A2 centre (1.6398, -64.7578) radius 1.75
  circle A3 centre (-115.8829, 1.4876) radius 1.75
  circle A4 centre (-41.6318, -51.3598) radius 1.5
  line L0 (-118.6011, -67.1556) -> (4.2373, -67.1556)
  line L1 (4.2373, -67.1556) -> (4.2373, 4.0256)
  line L2 (4.2373, 4.0256) -> (-118.6011, 4.0256)
  line L3 (-118.6011, 4.0256) -> (-118.6011, -67.1556)
  line L4 (-17.965, 0.2524) -> (-17.965, -29.1961)
  line L5 (-17.965, -29.1961) -> (-97.3004, -29.1961)
  line L6 (-97.3004, -29.1961) -> (-97.3004, 0.2524)
  line L7 (-97.3004, 0.2524) -> (-17.965, 0.2524)
  line L8 (-50, -40) -> (-45.0052, -40)
  line L9 (-45.0052, -40) -> (-45.0052, -32.6518)
  line L10 (-45.0052, -32.6518) -> (-50, -32.6518)
  line L11 (-50, -32.6518) -> (-50, -40)
  line L12 (-65, -40) -> (-69.9862, -40)
  line L13 (-69.9862, -40) -> (-69.9862, -32.6518)
  line L14 (-69.9862, -32.6518) -> (-65, -32.6518)
  line L15 (-65, -32.6518) -> (-65, -40)
  constraint horizontal L8
  constraint vertical L9
  constraint horizontal L10
  constraint vertical L11
  constraint horizontal L12
  constraint vertical L13
  constraint horizontal L14
  constraint vertical L15
extrude "Extrude57" add sketch "Sketch35" along normal blind 6 contours L8 L9 L10 L11 | L12 L13 L14 L15 bodies 10 in component "Case"
sketch "Sketch36" plane through (45.0052, 0, 0) normal (-1, 0, 0) x (0, -1, 0)
  line L0 (-40, 11) -> (-32.6518, 11)
  line L1 (-32.6518, 11) -> (-32.6518, 17)
  line L2 (-32.6518, 17) -> (-40, 17)
  line L3 (-40, 17) -> (-40, 11)
fillet "Fillet9" radius 3 2 edges at (47.5026, 40, 17) (47.5026, 32.6518, 17) on bodies 10 in component "Case"
fillet "Fillet10" radius 3 2 edges at (67.4931, 40, 17) (67.4931, 32.6518, 17) on bodies 10 in component "Case"
sketch "Sketch37" plane through (45.0052, 0, 0) normal (-1, 0, 0) x (0, -1, 0)
sketch "Sketch38" plane through (45.0052, 0, 0) normal (-1, 0, 0) x (0, -1, 0)
  arc A0 (-32.6518, 14) -> (-35.6518, 17) centre (-35.6518, 14) ccw
  line L0 (-35.6518, 17) -> (-37, 17)
  arc A1 (-37, 17) -> (-40, 14) centre (-37, 14) ccw
  line L1 (-40, 14) -> (-40, 11)
  line L2 (-40, 11) -> (-32.6518, 11)
  line L3 (-32.6518, 11) -> (-32.6518, 14)
  circle A2 centre (-36.3259, 13.8137) radius 1.82
extrude "Extrude58" cut sketch "Sketch38" against normal blind 40 contours A2 bodies 10 in component "Case"
component "Case" placed x (1, 0, 0) y (0, 1, 0) z (0, 0, 1) at (0, 0, 0)
named bodies: "PCB", "Battery", "Rough Clearance", "USB", "Front", "Back"
